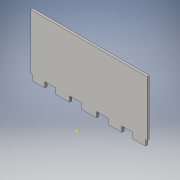
# Autodesk Inventor part: mcdave_ramp
Saved by Autodesk Inventor 2016 (Build 200138000, 138)
## iProperties
Created: 2017-11-27
Part Number: mcdave_ramp
Material: Generic
Document SubType Name: Modeling
Designer: student
Density: 1 g/cm^3
Appearance: Default
Author: student
Autodesk Inventor part; units mm, degrees
ref_plane "YZ Plane" through (0, 0, 0) normal (1, 0, 0) x (0, 1, 0)
ref_plane "XZ Plane" through (0, 0, 0) normal (0, 1, 0) x (-1, 0, 0)
ref_plane "XY Plane" through (0, 0, 0) normal (0, 0, 1) x (1, 0, 0)
sketch "Sketch1" plane through (0, 0, 0) normal (0, 0, 1) x (1, 0, 0)
  line L0 (-44.7811, 27.3777) -> (-44.7811, 21.678)
  line L1 (69.7802, 27.3777) -> (69.7802, 21.678)
  line L2 (69.7802, 27.3777) -> (69.7802, 21.678)
  line L3 (-44.7811, 21.678) -> (-31.9793, 21.678)
  line L4 (-31.9793, 27.3777) -> (-31.9793, 21.678)
  line L5 (-31.9793, 27.3777) -> (-31.9793, 21.678)
  line L6 (-20.8402, 21.678) -> (-20.8402, 27.3777)
  line L7 (-20.8402, 27.3777) -> (-20.8402, 21.678)
  line L8 (4.7205, 21.678) -> (4.7205, 27.3777)
  line L9 (4.7205, 27.3777) -> (4.7205, 21.678)
  line L10 (20.2786, 27.3777) -> (20.2786, 21.678)
  line L11 (20.2786, 27.3777) -> (20.2786, 21.678)
  line L12 (31.9768, 27.3777) -> (31.9768, 21.678)
  line L13 (45.8394, 27.3777) -> (45.8394, 21.678)
  line L14 (45.8394, 27.3777) -> (45.8394, 21.678)
  line L15 (56.9784, 21.678) -> (69.7802, 21.678)
  line L16 (56.9784, 27.3777) -> (56.9784, 21.678)
  line L17 (-6.9776, 27.3777) -> (-6.9776, 21.678)
  line L18 (-31.9793, 21.678) -> (-44.7811, 21.678)
  line L19 (-6.9776, 21.678) -> (-20.8402, 21.678)
  line L20 (20.2786, 21.678) -> (4.7205, 21.678)
  line L21 (69.7802, 21.678) -> (56.9784, 21.678)
  line L22 (45.8394, 21.678) -> (31.9768, 21.678)
  line L23 (-44.7811, 27.3777) -> (-44.7811, 83.2577)
  line L24 (-44.7811, 83.2577) -> (69.7802, 83.2577)
  line L25 (69.7802, 83.2577) -> (69.7802, 27.3777)
  line L26 (56.9784, 27.3777) -> (45.8394, 27.3777)
  line L27 (31.9768, 27.3777) -> (20.2786, 27.3777)
  line L28 (4.7205, 27.3777) -> (-6.9776, 27.3777)
  line L29 (-20.8402, 27.3777) -> (-31.9793, 27.3777)
  point P0 (0, 0)
  dimension "d0" = 55.88
  constraints: 60 end point, 12 collinear, 6 perpendicular, 4 vertical, 1 horizontal
  measures "d0" distance of L0.start L23.end
extrude "Extrusion1" add sketch "Sketch1" along normal blind 2.286
sketch "Sketch2" plane through (0, 0, 2.286) normal (0, 0, 1) x (1, 0, 0)
  line L0 (-31.9793, 21.678) -> (-31.9793, 27.3777) projected
  line L1 (-44.7811, 83.2577) -> (-44.7811, 21.678) projected
  line L2 (-44.7811, 27.3777) -> (-46.3559, 27.3777)
  line L3 (-44.7811, 83.2577) -> (-46.3559, 83.2577)
  line L4 (-46.3559, 83.2577) -> (-46.3559, 27.3777)
  line L5 (69.7802, 83.2577) -> (-44.7811, 83.2577) projected
  line L6 (69.7802, 27.3777) -> (71.355, 27.3777)
  line L7 (71.355, 83.2577) -> (71.355, 27.3777)
  line L8 (-44.7811, 83.2577) -> (-44.7811, 27.3777)
  line L9 (69.7802, 83.2577) -> (71.355, 83.2577)
  line L10 (69.7802, 21.678) -> (69.7802, 83.2577) projected
  line L11 (69.7802, 83.2577) -> (69.7802, 27.3777)
  point P0 (0, 0)
  dimension "d3" = 1.5748
  constraints: 16 end point, 2 collinear, 2 perpendicular, 1 horizontal, 1 parallel, 1 point on line
  measures "d3" distance of L2.start L2.end
extrude "Extrusion2" add sketch "Sketch2" against normal blind 2.286
sketch "Sketch3" plane through (0, 0, 2.286) normal (0, 0, 1) x (1, 0, 0)
  point P0 (0, 0)
body "Solid1"
